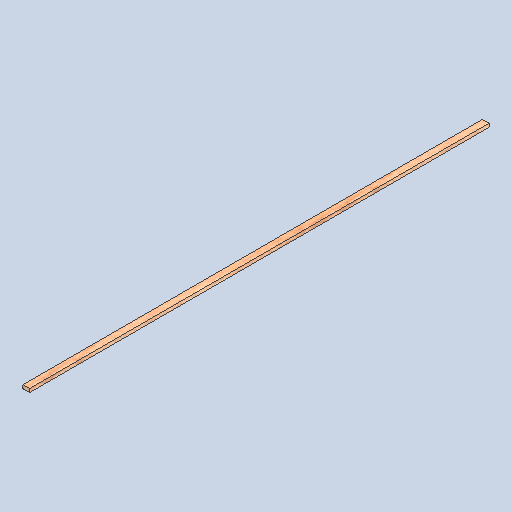
# Autodesk Inventor part: 2P.03.01.11.IM.FlapBottSpanBeam
Saved by Autodesk Inventor 2025.2 (Build 292293000, 293)
## iProperties
Created: 2025-01-07
Part Number: 2P.03.01.11.IM.FlapBottSpanBeam
Material: Wood (Birch)
Document SubType Name: Modeling
Designer: Imist
Density: 0.55 g/cm^3
Appearance: Birch - Natural Polished
Author: Imist
Autodesk Inventor part; units mm, degrees
ref_plane "YZ Plane" through (0, 0, 0) normal (1, 0, 0) x (0, 1, 0)
ref_plane "XZ Plane" through (0, 0, 0) normal (0, 1, 0) x (-1, 0, 0)
ref_plane "XY Plane" through (0, 0, 0) normal (0, 0, 1) x (1, 0, 0)
sketch "Sketch1" plane through (0, 0, 0) normal (0, 0, 1) x (1, 0, 0)
  line L0 (-11.9182, 1.5) -> (-6.2332, 1.5)
  line L1 (-6.2332, 1.5) -> (-6.2332, -1.5)
  line L2 (-6.2332, -1.5) -> (-11.9182, -1.5)
  line L3 (-11.9182, -1.5) -> (-11.9182, 1.5)
  line L4 (-11.9182, 1.5) -> (-6.2332, -1.5) construction
  line L5 (-6.2332, 1.5) -> (-11.9182, -1.5) construction
  point P0 (0, 0)
  point P1 (-9.0757, 0)
  dimension "d0" = 3
  dimension "d1" = 5.685
  constraints: 12 end point, 2 midpoint, 2 parallel, 1 horizontal, 1 perpendicular
  measures "d0" distance of L2.end L0.start
  measures "d1" distance of L0.start L0.end
extrude "Extrusion1" add sketch "Sketch1" along normal blind 393
body "Solid1"
